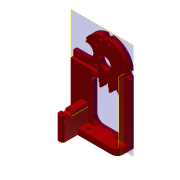
# Autodesk Inventor part: G004175_Cycl_marcoIzquierdoX
Saved by Autodesk Inventor 2015 SP2 (Build 190223200, 223)
## iProperties
Created: 2015-05-05
Part Number: G004175_Cycl_marcoIzquierdoX
Material: Genérico
Document SubType Name: Modeling
Designer: EDU
Density: 1 g/cm^3
Appearance: Suave - Rojo
Author: EDU
Autodesk Inventor part; units mm, degrees
ref_plane "YZ Plane" through (0, 0, 0) normal (1, 0, 0) x (0, 1, 0)
sketch "Boceto1" plane through (0, 0, 0) normal (0, 0, 1) x (1, 0, 0)
  line L0 (-49.75, 14.5) -> (49.75, 14.5)
  line L1 (49.75, 14.5) -> (49.75, -14.5)
  line L2 (49.75, -14.5) -> (-49.75, -14.5)
  line L3 (-49.75, -14.5) -> (-49.75, 14.5)
  point P0 (0, 0)
  point P1 (0, 14.5)
  point P2 (49.75, 0)
  dimension "d0" = 29
  dimension "d1" = 99.5
  constraints: 8 end point, 2 midpoint, 2 parallel, 1 horizontal, 1 horizontal alignment, 1 perpendicular, 1 vertical alignment
  measures "d0" distance of L0.end L1.end
  measures "d1" distance of L0.start L0.end
extrude "Extrusión1" add sketch "Boceto1" along normal blind 10
sketch "Boceto2" plane through (0, 0, 10) normal (0, 0, 1) x (1, 0, 0)
  line L0 (49.75, -14.5) -> (49.75, 14.5) projected
  line L1 (-49.75, 14.5) -> (49.75, 14.5)
  line L2 (49.75, 14.5) -> (49.75, 3.5)
  line L3 (49.75, 3.5) -> (-49.75, 3.5)
  line L4 (-49.75, 3.5) -> (-49.75, 14.5)
  point P0 (0, 0)
  dimension "d4" = 11
  constraints: 8 end point, 2 parallel, 1 horizontal, 1 perpendicular, 1 point on line
  measures "d4" distance of L1.end L2.end
extrude "Extrusión2" add sketch "Boceto2" along normal blind 144
sketch "Boceto3" plane through (-49.75, 3.5, 10) normal (0, -1, 0) x (1, 0, 0)
  line L0 (15, 76.5) -> (64.5, 76.5)
  line L1 (64.5, 76.5) -> (64.5, 0)
  line L2 (64.5, 0) -> (15, 0)
  line L3 (15, 0) -> (15, 76.5)
  line L4 (0, 0) -> (0, 144) projected
  point P0 (49.75, -10)
  point P1 (99.5, 0)
  dimension "d7" = 15
  dimension "d8" = 49.5
  dimension "d9" = 76.5
  constraints: 8 end point, 2 parallel, 1 horizontal, 1 horizontal alignment, 1 perpendicular
  measures "d7" distance between parallel lines of L4 L3
  measures "d8" distance of L0.start L0.end
  measures "d9" distance of L0.end L1.end
extrude "Extrusión3" cut sketch "Boceto3" against normal blind 154
fillet "Empalme1" radius 13 4 edges at (-34.75, 9, 10) (14.75, 9, 10) (-34.75, 9, 86.5) (14.75, 9, 86.5)
sketch "Boceto4" plane through (-49.75, 3.5, 154) normal (0, -1, 0) x (1, 0, 0)
  circle A0 centre (39.75, -40) radius 11.25
  line L0 (28, -67.5) -> (51.5, -67.5) projected
  point P0 (49.75, -154)
  point P1 (39.75, -67.5)
  dimension "d13" = 22.5
  dimension "d14" = 27.5
  constraints: 1 centre point, 1 midpoint, 1 vertical alignment
  measures "d13" diameter of A0
  measures "d14" distance from line of L0 A0.centre
extrude "Extrusión4" cut sketch "Boceto4" against normal blind 3
fillet "Empalme2" radius 10 2 edges at (49.75, -14.5, 5) (-49.75, -14.5, 5)
sketch "Boceto6" plane through (-49.75, 3.5, 154) normal (0, -1, 0) x (1, 0, 0)
  line L0 (0, -154) -> (99.5, -154) projected
  line L1 (69.5, -154) -> (80.5, -154)
  line L2 (80.5, -154) -> (80.5, -114)
  line L3 (80.5, -114) -> (69.5, -114)
  line L4 (69.5, -114) -> (69.5, -154)
  line L5 (64.5, -80.5) -> (64.5, -131) projected
  point P0 (49.75, -154)
  dimension "d21" = 5
  dimension "d22" = 40
  dimension "d23" = 11
  constraints: 8 end point, 2 parallel, 1 horizontal, 1 perpendicular, 1 point on line
  measures "d21" distance between parallel lines of L4 L5
  measures "d22" distance of L1.end L2.end
  measures "d23" distance of L2.end L3.end
extrude "Extrusión6" add sketch "Boceto6" along normal blind 44
fillet "Empalme3" radius 4 2 edges at (30.75, -40.5, 20) (19.75, -40.5, 20)
sketch "Boceto8" plane through (19.75, 3.5, 40) normal (0, 0, 1) x (1, 0, 0)
  arc A0 (0, -40) -> (4, -44) centre (4, -40) ccw projected
  line L0 (7, -44) -> (4, -44) projected
  arc A1 (7, -44) -> (11, -40) centre (7, -40) ccw projected
  line L1 (11, 0) -> (11, -40) projected
  line L2 (0, 0) -> (11, 0) projected
  line L3 (0, 0) -> (0, -40) projected
  circle A2 centre (5.5, -38.75) radius 1.75
  circle A3 centre (5.5, -24.25) radius 1.75
  line L4 (7, -44) -> (4, -44) projected
  point P0 (-19.75, -3.5)
  point P1 (5.5, -44)
  point P2 (5.5, -44)
  dimension "d33" = 3.5
  dimension "d34" = 3.5
  dimension "d35" = 5.25
  dimension "d36" = 14.5
  constraints: 2 centre point, 2 midpoint, 2 vertical alignment
  measures "d33" diameter of A2
  measures "d34" diameter of A3
  measures "d35" distance from line of L0 A2.centre
  measures "d36" distance of A2.centre A3.centre
extrude "Extrusión8" cut sketch "Boceto8" against normal blind 20 contours A2 | A3
sketch "Boceto9" plane through (30.75, 3.5, 40) normal (1, 0, 0) x (0, 0, -1)
  line L0 (40, -40) -> (0, -40) projected
  line L1 (40, -18) -> (40, -40) projected
  line L2 (30, -18) -> (40, -18) projected
  line L3 (30, 0) -> (30, -18) projected
  line L4 (0, 0) -> (30, 0) projected
  line L5 (0, 0) -> (0, -40) projected
  line L6 (0, 0) -> (0, -40) projected
  arc A0 (0, -35.5) -> (0, -27.5) centre (0, -31.5) ccw
  point P0 (40, -3.5)
  point P1 (0, -44)
  dimension "d39" = 8
  dimension "d40" = 12.5
  constraints: 2 point on circle, 2 point on line, 1 centre point, 1 vertical alignment
  measures "d39" distance of A0.start A0.end
  measures "d40" distance of point (0, -44) A0.centre
extrude "Extrusión9" cut sketch "Boceto9" against normal through all contours L5 A0
sketch "Boceto10" plane through (30.75, 3.5, 40) normal (1, 0, 0) x (0, 0, -1)
  arc A0 (0, -35.5) -> (0, -27.5) centre (0, -31.5) ccw projected
  line L0 (0, -35.5) -> (0, -40) projected
  line L1 (40, -40) -> (0, -40) projected
  line L2 (40, -18) -> (40, -40) projected
  line L3 (30, -18) -> (40, -18) projected
  line L4 (30, 0) -> (30, -18) projected
  line L5 (0, 0) -> (30, 0) projected
  line L6 (0, 0) -> (0, -27.5) projected
  circle A1 centre (25, -5) radius 5
  line L7 (30, 0) -> (-114, 0) projected
  line L8 (30, -8) -> (30, 0) projected
  point P0 (40, -3.5)
  dimension "d43" = 10
  constraints: 2 tangent, 1 centre point
  measures "d43" diameter of A1
extrude "Extrusión10" cut sketch "Boceto10" against normal through all contours A1
sketch "Boceto11" plane through (-49.75, 14.5, 0) normal (0, 1, 0) x (1, 0, 0)
  line L0 (51.5, -86.5) -> (28, -86.5) projected
  line L1 (50.5, -86.5) -> (50.5, -81.25)
  line L2 (50.5, -81.25) -> (49.25, -80)
  line L3 (49.25, -80) -> (49.25, -74)
  line L4 (49.25, -74) -> (46.75, -74)
  line L5 (46.75, -74) -> (46.75, -80)
  line L6 (46.75, -80) -> (45.5, -81.25)
  line L7 (45.5, -81.25) -> (45.5, -86.5)
  line L8 (28, -86.5) -> (51.5, -86.5) projected
  line L9 (34, -86.5) -> (34, -81.25)
  line L10 (32.75, -80) -> (32.75, -74)
  line L11 (32.75, -74) -> (30.25, -74)
  line L12 (30.25, -74) -> (30.25, -80)
  line L13 (29, -81.25) -> (29, -86.5)
  line L14 (34, -81.25) -> (32.75, -80)
  line L15 (30.25, -80) -> (29, -81.25)
  point P0 (49.75, 0)
  point P1 (39.75, -86.5)
  dimension "d46" = 12.5
  dimension "d47" = 6
  dimension "d48" = 2.5
  dimension "d49" = 2.5
  dimension "d50" = 5
  dimension "d51" = 5
  dimension "d52" = 21.5
  dimension "d53" = 5.75
  constraints: 28 end point, 8 perpendicular, 6 horizontal alignment, 6 point on line, 2 equal length, 2 parallel, 1 midpoint, 1 vertical
  measures "d46" distance between parallel lines of L8 L11
  measures "d47" distance of L10.start L10.end
  measures "d48" distance of L10.end L11.end
  measures "d49" distance of L3.end L4.end
  measures "d50" distance between parallel lines of L13 L9
  measures "d51" distance between parallel lines of L1 L7
  measures "d52" distance between parallel lines of L13 L1
  measures "d53" distance from line of L7 point (39.75, -86.5)
extrude "Extrusión11" add sketch "Boceto11" against normal up to surface (11 mm away) contours L0 L13 L15 L12 L11 L10 L14 L9
ref_plane "Plano de trabajo1" through (-10, 3.5, 73.5) normal (1, 0, 0) x (0, 0, -1)
mirror "Simetría1" about plane through (-10, 3.5, 73.5) normal (1, 0, 0) of "Extrusión11"
sketch "Boceto12" plane through (-49.75, 3.5, 10) normal (0, -1, 0) x (1, 0, 0)
  line L0 (0, -10) -> (0, 144) projected
  arc A0 (75.9203, 120.4855) -> (0, 104) centre (39.75, 104) ccw
  line L1 (0, 0) -> (0, 144) projected
  line L2 (10, -10) -> (0, -10) projected
  circle A1 centre (39.75, 104) radius 11.25 projected
  line L3 (75.9203, 120.4855) -> (99.5, 68.75)
  line L4 (99.5, 68.75) -> (99.5, 156.8559)
  line L5 (99.5, 156.8559) -> (0, 156.8559)
  line L6 (0, 156.8559) -> (0, 104)
  line L7 (99.5, -10) -> (89.5, -10) projected
  point P0 (49.75, -10)
  dimension "d57" = 78.75
  constraints: 8 end point, 3 tangent, 2 coincident, 2 perpendicular, 2 point on circle, 1 centre point, 1 point on line, 1 vertical, 1 vertical alignment
  measures "d57" distance from line of L7 L3.end
extrude "Extrusión12" cut sketch "Boceto12" against normal through all contours L0 L6 L5 L4 L3 A0
sketch "Boceto13" plane through (0, 0, 0) normal (0, 0, -1) x (-1, 0, 0)
  line L0 (-49.75, 14.5) -> (-49.75, -4.5) projected
  line L1 (49.75, 14.5) -> (-49.75, 14.5) projected
  point P0 (0, 0)
  point P1 (-40.25, -5.5)
  point P2 (-8.75, -5.5)
  point P3 (41.25, -5.5)
  dimension "d60" = 50
  dimension "d61" = 31.5
  dimension "d62" = 9.5
  dimension "d63" = 20
  constraints: 2 horizontal alignment
  measures "d60" distance of point (41.25, -5.5) point (-8.75, -5.5)
  measures "d61" distance of point (-8.75, -5.5) point (-40.25, -5.5)
  measures "d62" distance from line of L0 point (-40.25, -5.5)
  measures "d63" distance from line of L1 point (-40.25, -5.5)
hole "Agujero1" at (40.25, -5.5, 0) at (8.75, -5.5, 0) at (-41.25, -5.5, 0) direction (0, 0, 1) diameter 3.5 end through all
sketch "Boceto16" plane through (0, 0, 10) normal (0, 0, 1) x (1, 0, 0)
  circle A0 centre (-41.25, -5.5) radius 1.75 projected
  circle A1 centre (8.75, -5.5) radius 1.75 projected
  circle A2 centre (40.25, -5.5) radius 1.75 projected
  line L0 (-39.4501, -2.3825) -> (-37.6502, -5.5)
  line L1 (-37.6502, -5.5) -> (-39.4501, -8.6175)
  line L2 (-39.4501, -8.6175) -> (-43.0499, -8.6175)
  line L3 (-43.0499, -8.6175) -> (-44.8498, -5.5)
  line L4 (-44.8498, -5.5) -> (-43.0499, -2.3825)
  line L5 (-43.0499, -2.3825) -> (-39.4501, -2.3825)
  line L6 (10.5499, -2.3825) -> (12.3498, -5.5)
  line L7 (12.3498, -5.5) -> (10.5499, -8.6175)
  line L8 (10.5499, -8.6175) -> (6.9501, -8.6175)
  line L9 (6.9501, -8.6175) -> (5.1502, -5.5)
  line L10 (5.1502, -5.5) -> (6.9501, -2.3825)
  line L11 (6.9501, -2.3825) -> (10.5499, -2.3825)
  line L12 (42.0499, -2.3825) -> (43.8498, -5.5)
  line L13 (43.8498, -5.5) -> (42.0499, -8.6175)
  line L14 (42.0499, -8.6175) -> (38.4501, -8.6175)
  line L15 (38.4501, -8.6175) -> (36.6502, -5.5)
  line L16 (36.6502, -5.5) -> (38.4501, -2.3825)
  line L17 (38.4501, -2.3825) -> (42.0499, -2.3825)
  point P0 (0, 0)
  dimension "d77" = 6.235
  constraints: 36 end point, 3 coincident, 3 horizontal, 2 horizontal alignment, 39 other
  measures "d77" distance between parallel lines of L2 L5
extrude "Extrusión15" cut sketch "Boceto16" against normal blind 2.79
ref_plane "Plano de trabajo2" through (-49.75, 9, 10) normal (0, -1, 0) x (1, 0, 0)
ref_plane "Plano de trabajo3" through (-10, 3.5, 153.75) normal (0, 0, 1) x (1, 0, 0)
sketch "Boceto17" plane through (-10, 3.5, 153.75) normal (0, 0, 1) x (1, 0, 0)
  line L0 (-39.75, 11) -> (36.1703, 11) construction
  line L1 (-39.75, 11) -> (-39.75, 0) projected
  line L2 (36.1703, 0) -> (-39.75, 0) projected
  line L3 (36.1703, 0) -> (36.1703, 11) construction
  line L4 (79.65, 5.5) -> (-59.65, 5.5) projected
  circle A0 centre (-7.25, 5.5) radius 1.875
  circle A1 centre (7.25, 5.5) radius 1.875
  line L5 (11.25, 0) -> (-11.25, 0) projected
  point P0 (10, -3.5)
  point P1 (-24.75, 0)
  point P2 (24.75, 0)
  dimension "d80" = 3.75
  dimension "d81" = 3.75
  dimension "d82" = 14.5
  dimension "d88" = 17.5
  dimension "d89" = 17.5
  constraints: 2 centre point, 2 point on line
  measures "d80" diameter of A1
  measures "d81" diameter of A0
  measures "d82" distance of A0.centre A1.centre
  measures "d88" horizontal distance of point (-24.75, 0) A0.centre
  measures "d89" horizontal distance of A1.centre point (24.75, 0)
extrude "Extrusión16" cut sketch "Boceto17" against normal blind 15
sketch "Boceto14" plane through (-49.75, 3.5, 10) normal (0, -1, 0) x (1, 0, 0)
  circle A0 centre (0, 104) radius 4.3
  point P0 (49.75, -10)
  dimension "d71" = 8.6
  constraints: 1 centre point
  measures "d71" diameter of A0
extrude "Extrusión13" cut sketch "Boceto14" against normal blind 20
sketch "Boceto15" plane through (-49.75, 3.5, 10) normal (0, -1, 0) x (1, 0, 0)
  arc A0 (75.9203, 120.4855) -> (0.2326, 108.2937) centre (39.75, 104) ccw projected
  circle A1 centre (39.75, 143.75) radius 4.3
  point P0 (49.75, -10)
  dimension "d74" = 8.6
  constraints: 1 centre point, 1 point on circle, 1 vertical alignment
  measures "d74" diameter of A1
extrude "Extrusión14" cut sketch "Boceto15" against normal blind 20
sketch "Boceto18" plane through (-49.75, -4.5, 0) normal (-1, 0, 0) x (0, 0, 1)
  circle A0 centre (121.2774, 13.5) radius 1.875
  circle A1 centre (106.7774, 13.5) radius 1.875
  line L0 (118.2937, 19) -> (118.2937, 8) projected
  line L1 (118.2937, 19) -> (118.2937, 8) projected
  line L2 (109.7, 19) -> (118.2937, 19) projected
  line L3 (109.7, 8) -> (109.7, 19) projected
  line L4 (118.2937, 8) -> (109.7, 8) projected
  line L5 (153.5174, 19) -> (153.5174, 8) projected
  line L6 (130.4855, 8) -> (153.5174, 8) projected
  line L7 (130.4855, 8) -> (130.4855, 19) projected
  line L8 (153.5174, 19) -> (130.4855, 19) projected
  point P0 (0, 4.5)
  point P1 (118.2937, 13.5)
  dimension "d90" = 3.75
  dimension "d91" = 3.75
  dimension "d92" = 14.5
  constraints: 2 centre point, 2 horizontal alignment, 1 midpoint, 1 other
  measures "d90" diameter of A0
  measures "d91" diameter of A1
  measures "d92" distance of A1.centre A0.centre
extrude "Extrusión17" cut sketch "Boceto18" against normal blind 15 contours A0 | A1
mirror "Simetría2" about plane through (-49.75, 9, 10) normal (0, -1, 0) of "Extrusión6", "Extrusión8", "Extrusión9", "Extrusión10", "Empalme3", "Extrusión15", "Extrusión1", "Agujero1", "Empalme2"
sketch "Boceto19" plane through (49.75, -4.5, 10) normal (1, 0, 0) x (0, 0, -1)
  line L0 (-30, 8) -> (-30, -19.5) projected
  line L1 (0, 8) -> (-68.75, 8) projected
  line L2 (-30, 8) -> (10, 8)
  line L3 (10, 8) -> (10, -42)
  line L4 (10, -42) -> (-30, -42)
  line L5 (-30, -42) -> (-30, 8)
  point P0 (10, 4.5)
  dimension "d95" = 50
  dimension "d96" = 40
  constraints: 8 end point, 2 parallel, 1 horizontal, 1 perpendicular
  measures "d95" distance of L4.end L0.start
  measures "d96" distance of L3.end L4.end
extrude "Extrusión18" cut sketch "Boceto19" against normal through all
sketch "Boceto21" plane through (-10, 6.5, 114) normal (0, -1, 0) x (1, 0, 0)
  circle A0 centre (0, 0) radius 11.25 projected
  circle A1 centre (0, 0) radius 10.3
  point P0 (10, -114)
  dimension "d101" = 20.6
  constraints: 1 centre point, 1 coincident
  measures "d101" diameter of A1
extrude "Extrusión20" cut sketch "Boceto21" against normal blind 14 contours A1
sketch "Boceto22" plane through (-49.75, 14.5, 10) normal (0, 1, 0) x (1, 0, 0)
  line L0 (94.65, -125.25) -> (52.15, -125.25)
  line L1 (52.15, -125.25) -> (52.15, -82.75)
  line L2 (52.15, -82.75) -> (94.65, -82.75)
  line L3 (94.65, -82.75) -> (94.65, -125.25)
  circle A0 centre (39.75, -104) radius 10.3 projected
  point P0 (49.75, 10)
  point P1 (50.05, -104)
  point P2 (52.15, -104)
  dimension "d104" = 42.5
  dimension "d105" = 42.5
  dimension "d129" = 2.1
  constraints: 8 end point, 3 horizontal alignment, 2 parallel, 1 horizontal, 1 midpoint, 1 perpendicular, 1 other
  measures "d104" distance of L1.end L2.end
  measures "d105" distance of L0.end L1.end
  measures "d129" distance from line of L1 point (50.05, -104)
extrude "Extrusión21" cut sketch "Boceto22" against normal blind 5 contours L0 L1 L2 L3
sketch "Boceto23" plane through (-49.75, 14.5, 10) normal (0, 1, 0) x (1, 0, 0)
  line L0 (73.3432, -125.25) -> (52.15, -125.25) projected
  line L1 (52.15, -125.25) -> (52.15, -82.75) projected
  line L2 (52.15, -82.75) -> (93.1192, -82.75) projected
  line L3 (93.1192, -82.75) -> (99.5, -68.75) projected
  line L4 (99.5, 0) -> (99.5, -68.75) projected
  line L5 (99.5, 0) -> (80.5, 0) projected
  line L6 (80.5, 0) -> (80.5, -5) projected
  line L7 (80.5, -5) -> (80.5, -30) projected
  line L8 (80.5, -30) -> (69.5, -30) projected
  line L9 (69.5, -30) -> (69.5, -5) projected
  line L10 (69.5, -5) -> (69.5, 0) projected
  line L11 (69.5, 0) -> (51.5, 0) projected
  arc A0 (64.5, -13) -> (51.5, 0) centre (51.5, -13) ccw projected
  line L12 (64.5, -13) -> (64.5, -63.5) projected
  arc A1 (51.5, -76.5) -> (64.5, -63.5) centre (51.5, -63.5) ccw projected
  line L13 (51.5, -76.5) -> (50.5, -76.5) projected
  line L14 (50.5, -71.25) -> (50.5, -76.5) projected
  line L15 (49.25, -70) -> (50.5, -71.25) projected
  line L16 (49.25, -64) -> (49.25, -70) projected
  line L17 (46.75, -64) -> (49.25, -64) projected
  line L18 (46.75, -70) -> (46.75, -64) projected
  line L19 (45.5, -71.25) -> (46.75, -70) projected
  line L20 (45.5, -76.5) -> (45.5, -71.25) projected
  line L21 (45.5, -76.5) -> (34, -76.5) projected
  line L22 (34, -76.5) -> (34, -71.25) projected
  line L23 (34, -71.25) -> (32.75, -70) projected
  line L24 (32.75, -70) -> (32.75, -64) projected
  line L25 (32.75, -64) -> (30.25, -64) projected
  line L26 (30.25, -64) -> (30.25, -70) projected
  line L27 (30.25, -70) -> (29, -71.25) projected
  line L28 (29, -71.25) -> (29, -76.5) projected
  line L29 (29, -76.5) -> (28, -76.5) projected
  arc A2 (15, -63.5) -> (28, -76.5) centre (28, -63.5) ccw projected
  line L30 (15, -63.5) -> (15, -13) projected
  arc A3 (28, 0) -> (15, -13) centre (28, -13) ccw projected
  line L31 (28, 0) -> (0, 0) projected
  line L32 (0, 0) -> (0, -99.7) projected
  arc A4 (0.2326, -108.2937) -> (0, -99.7) centre (0, -104) ccw projected
  arc A5 (0.2326, -108.2937) -> (35.4563, -143.5174) centre (39.75, -104) ccw projected
  arc A6 (44.0437, -143.5174) -> (35.4563, -143.5174) centre (39.75, -143.75) ccw projected
  arc A7 (44.0437, -143.5174) -> (73.3432, -125.25) centre (39.75, -104) ccw projected
  circle A8 centre (39.75, -104) radius 10.3 projected
  line L33 (99.5, -68.75) -> (93.1192, -68.75)
  line L34 (93.1192, -68.75) -> (93.1192, -82.75)
  line L35 (93.1192, -82.75) -> (99.5, -82.75)
  line L36 (99.5, -82.75) -> (99.5, -68.75)
  point P0 (49.75, 10)
  constraints: 8 end point, 2 parallel, 1 horizontal, 1 perpendicular
extrude "Extrusión22" add sketch "Boceto23" against normal blind 11 contours L3 L36 L35
sketch "Boceto24" plane through (-49.75, 9.5, 10) normal (0, 1, 0) x (1, 0, 0)
  arc A0 (73.3432, -125.25) -> (75.9203, -120.4855) centre (39.75, -104) ccw projected
  line L0 (93.1192, -82.75) -> (75.9203, -120.4855) projected
  line L1 (52.15, -82.75) -> (93.1192, -82.75) projected
  line L2 (52.15, -125.25) -> (52.15, -82.75) projected
  line L3 (73.3432, -125.25) -> (52.15, -125.25) projected
  line L4 (99.5, -82.75) -> (84.5, -82.75)
  line L5 (84.5, -82.75) -> (84.5, -92.75)
  line L6 (84.5, -92.75) -> (99.5, -92.75)
  line L7 (99.5, -92.75) -> (99.5, -82.75)
  point P0 (49.75, 10)
  dimension "d110" = 15
  dimension "d111" = 10
  constraints: 8 end point, 2 parallel, 1 horizontal, 1 perpendicular
  measures "d110" distance of L6.end L5.end
  measures "d111" distance of L5.end L4.end
extrude "Extrusión23" add sketch "Boceto24" against normal blind 6 contours L6 L5 L1 L0 | L0 L4 L7 L6
sketch "Boceto25" plane through (-49.75, 9.5, 10) normal (0, 1, 0) x (1, 0, 0)
  line L0 (52.15, -82.75) -> (99.5, -82.75) projected
  line L1 (52.15, -125.25) -> (52.15, -82.75) projected
  line L2 (73.3432, -125.25) -> (52.15, -125.25) projected
  arc A0 (73.3432, -125.25) -> (75.9203, -120.4855) centre (39.75, -104) ccw projected
  line L3 (88.5614, -92.75) -> (75.9203, -120.4855) projected
  line L4 (88.5614, -92.75) -> (99.5, -92.75) projected
  line L5 (99.5, -92.75) -> (99.5, -82.75) projected
  arc A1 (75.7378, -92.8503) -> (75.825, -115.15) centre (75.825, -104) ccw
  line L6 (52.15, -125.25) -> (52.15, -82.75) projected
  line L7 (52.15, -82.75) -> (99.5, -82.75) projected
  line L8 (75.7378, -92.8503) -> (88.5614, -92.75)
  line L9 (75.825, -115.15) -> (78.3521, -115.15)
  line L10 (78.3521, -115.15) -> (88.5614, -92.75)
  point P0 (49.75, 10)
  point P1 (52.15, -104)
  point P2 (75.825, -82.75)
  point P3 (75.825, -82.75)
  point P4 (75.825, -82.75)
  point P5 (66.85, -110.616)
  dimension "d114" = 22.3
  dimension "d127" = 32.65
  constraints: 6 end point, 4 midpoint, 3 point on circle, 2 tangent, 1 centre point, 1 coincident, 1 collinear, 1 horizontal, 1 horizontal alignment, 1 point on line, 1 vertical alignment
  measures "d114" diameter of A1
  measures "d127" distance from line of L5 point (66.85, -110.616)
extrude "Extrusión25" cut sketch "Boceto25" against normal blind 6 contours L3 L9 A1 L8
sketch "Boceto27" plane through (-49.75, 9.5, 10) normal (0, 1, 0) x (1, 0, 0)
  line L0 (78.3521, -115.15) -> (75.825, -115.15) projected
  arc A0 (75.7378, -92.8503) -> (75.825, -115.15) centre (75.825, -104) ccw projected
  line L1 (75.7378, -92.8503) -> (88.5614, -92.75) projected
  line L2 (88.5614, -92.75) -> (99.5, -92.75) projected
  line L3 (99.5, -92.75) -> (99.5, -82.75) projected
  line L4 (52.15, -82.75) -> (99.5, -82.75) projected
  line L5 (52.15, -125.25) -> (52.15, -82.75) projected
  line L6 (73.3432, -125.25) -> (52.15, -125.25) projected
  arc A1 (73.3432, -125.25) -> (75.9203, -120.4855) centre (39.75, -104) ccw projected
  line L7 (78.3521, -115.15) -> (75.9203, -120.4855) projected
  arc A2 (63.85, -121.45) -> (63.85, -117.65) centre (63.85, -119.55) ccw
  arc A3 (57.85, -117.65) -> (57.85, -121.45) centre (57.85, -119.55) ccw
  line L8 (63.85, -121.45) -> (57.85, -121.45)
  line L9 (57.85, -117.65) -> (63.85, -117.65)
  arc A4 (63.85, -90.45) -> (63.85, -86.65) centre (63.85, -88.55) ccw
  arc A5 (57.85, -86.65) -> (57.85, -90.45) centre (57.85, -88.55) ccw
  line L10 (63.85, -90.45) -> (57.85, -90.45)
  line L11 (57.85, -86.65) -> (63.85, -86.65)
  arc A6 (93.95, -121.45) -> (93.95, -117.65) centre (93.95, -119.55) ccw
  arc A7 (87.95, -117.65) -> (87.95, -121.45) centre (87.95, -119.55) ccw
  line L12 (93.95, -121.45) -> (87.95, -121.45)
  line L13 (87.95, -117.65) -> (93.95, -117.65)
  arc A8 (93.95, -90.45) -> (93.95, -86.65) centre (93.95, -88.55) ccw
  arc A9 (87.95, -86.65) -> (87.95, -90.45) centre (87.95, -88.55) ccw
  line L14 (93.95, -90.45) -> (87.95, -90.45)
  line L15 (87.95, -86.65) -> (93.95, -86.65)
  point P0 (49.75, 10)
  dimension "d132" = 3.8
  dimension "d133" = 3.8
  dimension "d134" = 6
  dimension "d135" = 5.7
  dimension "d136" = 5.7
  dimension "d139" = 31
  dimension "d142" = 30.1
  constraints: 16 end point, 16 point on circle, 8 centre point, 3 tangent, 1 horizontal, 1 horizontal alignment, 1 parallel, 1 vertical, 30 other
  measures "d132" diameter of A2
  measures "d133" diameter of A3
  measures "d134" distance of L8.start L8.end
  measures "d135" distance from line of L6 A3.centre
  measures "d136" distance from line of L5 A3.centre
  measures "d139" distance of L9.start L11.start
  measures "d142" distance of L9.start L13.start
extrude "Extrusión26" cut sketch "Boceto27" against normal through all contours L8 A3 L9 A2 | L10 A5 L11 A4 | L14 A9 L15 A8
sketch "Boceto28" plane through (19.75, 14.5, 40) normal (-1, 0, 0) x (0, 0, 1)
  arc A0 (-25, 0) -> (-30, 5) centre (-25, 5) ccw projected
  arc A1 (-30, 5) -> (-25, 0) centre (-25, 5) ccw projected
  point P0 (-40, -14.5)
extrude "Extrusión27" add sketch "Boceto28" against normal up to surface (11 mm away)
ref_plane "Plano de trabajo4" through (19.75, 42, 33.79) normal (0, 0, 1) x (1, 0, 0)
sketch "Boceto29" plane through (19.75, 42, 33.79) normal (0, 0, 1) x (1, 0, 0)
  circle A0 centre (5.5, 11.25) radius 1.75 projected
  circle A1 centre (5.5, -3.25) radius 1.75 projected
  line L0 (9.0998, 11.25) -> (7.2999, 8.1325)
  line L1 (7.2999, 8.1325) -> (3.7001, 8.1325)
  line L2 (3.7001, 14.3675) -> (7.2999, 14.3675)
  line L3 (7.2999, 14.3675) -> (9.0998, 11.25)
  line L4 (9.0998, -3.25) -> (7.2999, -6.3675)
  line L5 (7.2999, -6.3675) -> (3.7001, -6.3675)
  line L6 (3.7001, -0.1325) -> (7.2999, -0.1325)
  line L7 (7.2999, -0.1325) -> (9.0998, -3.25)
  line L8 (3.7001, 14.3675) -> (-0.5, 14.3675)
  line L9 (-0.5, 14.3675) -> (-0.5, 8.1325)
  line L10 (-0.5, 8.1325) -> (3.7001, 8.1325)
  line L11 (3.7001, -0.1325) -> (-0.5, -0.1325)
  line L12 (-0.5, -0.1325) -> (-0.5, -6.3675)
  line L13 (-0.5, -6.3675) -> (3.7001, -6.3675)
  point P0 (-19.75, -42)
  dimension "d150" = 6.235
  dimension "d151" = 6.235
  dimension "d152" = 6
  constraints: 28 end point, 3 horizontal, 3 perpendicular, 2 coincident, 2 point on line, 1 parallel, 16 other
  measures "d150" distance between parallel lines of L5 L6
  measures "d151" distance between parallel lines of L2 L1
  measures "d152" distance from line of A1.centre L12
extrude "Extrusión28" cut sketch "Boceto29" against normal blind 2.9
ref_plane "Plano de trabajo5" through (-10, 3.5, 147.54) normal (0, 0, 1) x (1, 0, 0)
sketch "Boceto30" plane through (-10, 3.5, 147.54) normal (0, 0, 1) x (1, 0, 0)
  circle A0 centre (7.25, 5.5) radius 1.875 projected
  circle A1 centre (-7.25, 5.5) radius 1.875 projected
  line L0 (7.25, 1.9002) -> (4.1325, 3.7001)
  line L1 (4.1325, 3.7001) -> (4.1325, 7.2999)
  line L2 (10.3675, 7.2999) -> (10.3675, 3.7001)
  line L3 (10.3675, 3.7001) -> (7.25, 1.9002)
  line L4 (-7.25, 1.9002) -> (-10.3675, 3.7001)
  line L5 (-10.3675, 3.7001) -> (-10.3675, 7.2999)
  line L6 (-4.1325, 7.2999) -> (-4.1325, 3.7001)
  line L7 (-4.1325, 3.7001) -> (-7.25, 1.9002)
  line L8 (10.3675, 7.2999) -> (10.3675, 11.5)
  line L9 (10.3675, 11.5) -> (4.1325, 11.5)
  line L10 (4.1325, 11.5) -> (4.1325, 7.2999)
  line L11 (-4.1325, 7.2999) -> (-4.1325, 11.5)
  line L12 (-4.1325, 11.5) -> (-10.3675, 11.5)
  line L13 (-10.3675, 11.5) -> (-10.3675, 7.2999)
  point P0 (10, -3.5)
  dimension "d156" = 6.235
  dimension "d157" = 6.235
  dimension "d158" = 6
  constraints: 28 end point, 3 perpendicular, 3 vertical, 2 coincident, 2 point on line, 1 parallel, 1 vertical alignment, 16 other
  measures "d156" distance between parallel lines of L1 L2
  measures "d157" distance of L4.end L6.end
  measures "d158" distance from line of L9 A0.centre
extrude "Extrusión29" cut sketch "Boceto30" against normal blind 2.85
ref_plane "Plano de trabajo6" through (-43.54, 3.5, 109.7) normal (-1, 0, 0) x (0, 0, 1)
sketch "Boceto31" plane through (-43.54, 3.5, 109.7) normal (-1, 0, 0) x (0, 0, 1)
  circle A0 centre (11.5774, 5.5) radius 1.875 projected
  circle A1 centre (-2.9226, 5.5) radius 1.875 projected
  line L0 (11.5774, 1.9002) -> (8.4599, 3.7001)
  line L1 (8.4599, 3.7001) -> (8.4599, 7.2999)
  line L2 (14.6949, 7.2999) -> (14.6949, 3.7001)
  line L3 (14.6949, 3.7001) -> (11.5774, 1.9002)
  line L4 (-2.9226, 1.9002) -> (-6.0401, 3.7001)
  line L5 (-6.0401, 3.7001) -> (-6.0401, 7.2999)
  line L6 (0.1949, 7.2999) -> (0.1949, 3.7001)
  line L7 (0.1949, 3.7001) -> (-2.9226, 1.9002)
  line L8 (14.6949, 7.2999) -> (14.6949, 11.5)
  line L9 (14.6949, 11.5) -> (8.4599, 11.5)
  line L10 (8.4599, 11.5) -> (8.4599, 7.2999)
  line L11 (0.1949, 7.2999) -> (0.1949, 11.5)
  line L12 (0.1949, 11.5) -> (-6.0401, 11.5)
  line L13 (-6.0401, 11.5) -> (-6.0401, 7.2999)
  point P0 (-109.7, -3.5)
  dimension "d162" = 6.235
  dimension "d163" = 6.235
  dimension "d164" = 6
  constraints: 28 end point, 2 coincident, 2 collinear, 2 point on line, 2 vertical alignment, 1 parallel, 1 perpendicular, 1 vertical, 16 other
  measures "d162" distance between parallel lines of L5 L6
  measures "d163" distance between parallel lines of L1 L2
  measures "d164" distance from line of L12 A1.centre
extrude "Extrusión30" cut sketch "Boceto31" against normal blind 2.85
chamfer "Chaflán1" distance 0.8 angle 30 1 edges at (-21.25, 3.5, 114) measured on face at (1.2135, 5.5, 113.0948)
fillet "Empalme4" radius 0.5 2 edges at (-49.5174, 9, 118.2937) (-49.75, 9, 109.7)
fillet "Empalme5" radius 0.5 2 edges at (-14.2937, 9, 153.5174) (-5.7063, 9, 153.5174)
equation "\"d105\" = d104"
